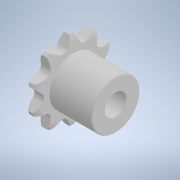
# Autodesk Inventor part: 25B10_()
Saved by Autodesk Inventor 2021 (Build 250183000, 183)
## iProperties
Created: 2025-03-15
Part Number: 25B10_()
Material: Generic
Catalog Web Link: www.cadenas.de
Description: K25B-Un-finished
Vendor: KANA
Document SubType Name: Modeling
Designer: psAdmin
Manufacturer: KANA
Mass: 2.29854 g
Surface Area: 15.9222 cm^2
Volume: 2.29854 cm^3
Density: 1 g/cm^3
Appearance: PSOLRGB-175-175-175
Category: PARTsolutions
Company: KANA
Title: K25B10
Author: Cadenas PARTsolutions
Comments: Un-finished
PSOL_IDENT_0: {$CADENAS_DATA/23d-libs/kana/sprockets/chain_no_25/un_finished_sprocket_steel/b_type/k25b.prj},157 {
PSOL_IDENT_1: VTYP=3D},{NB=25B10_()},{LINA=K25B10},{NN=K25B},{DATE=27.06.2023 01:46:12},{GEOMDATE=02.10.2020 05:05
PSOL_IDENT_2: :35},{VERSION=},{LINEID=10},{WBVAR=SURFT},{WBNUMERIC=}  {NB=25B10_()},{LINA=K25B10},{KT=DUMMY},{ORDE
PSOL_IDENT_3: RNO=K25B10},{TYPE=K25B},{NOT=10},{NOTX=10.000},{DP=20.55},{DO=23},{DC=17.25},{DC2=17.25},{T=2.8},{DR=
PSOL_IDENT_4: 3.3},{MAT=None},{MATC=},{SHAPE=C : Cutting type},{SHAPENB=C},{SD=6},{SURFT=},{SURFTNB=},{BD=14},{BL=
PSOL_IDENT_5: 15},{GD=0},{GDX=0},{S=0},{X=0},{VS=0},{SVDEL1=12},{SVDEL4=4},{SVDEL5=52},{DCX2=0},{CAUTION=The tooth
PSOL_IDENT_6: profile in the CAD models differ from the actual shape.}
NB: 25B10_()
NN: K25B
NT: Un-finished
NBSYN: 25B$NOT._($SURFT.)
LINA: K25B10
CATALOG: KANA
TYPE: K25B
NOT: 10
DP: 20.55
DO: 23
DC: 17.25
DC2: 17.25
T: 2.8
SHAPE: C : Cutting type
SD: 6
SURFT: No symbol : No
CAUTION: The tooth profile in the CAD models differ from the actual shape.
SUPPLIER: KANA
ARTICLENO: 25B10_()
BOMINFO: K25B10
CREATOR: CADENAS GmbH
Autodesk Inventor part; units mm, degrees
sketch "Sketch_4" plane through (0, 0, 0) normal (0, 0, 1) x (1, 0, 0)
  line L0 (15, 0) -> (0, 0)
  line L1 (0, 3.198) -> (0.198, 3)
  line L2 (0.198, 3) -> (14.802, 3)
  line L3 (14.802, 3) -> (15, 3.198)
  line L4 (15, 3.198) -> (15, 6.802)
  line L5 (15, 6.802) -> (14.802, 7)
  line L6 (14.802, 7) -> (2.8, 7)
  line L7 (2.8, 7) -> (2.8, 9.8274)
  arc A0 (2.8, 9.8274) -> (2.1, 11.5) centre (-0.477, 9.4387) ccw
  line L8 (2.1, 11.5) -> (0.7, 11.5)
  arc A1 (0.7, 11.5) -> (0, 9.8274) centre (3.277, 9.4387) ccw
  line L9 (0, 9.8274) -> (0, 3.198)
  constraints: 20 end point, 4 point on circle, 2 centre point
revolve "Revolution1" add sketch "Sketch_4" angle 360 about axis through (15, 0, 0) along (1, 0, 0)
sketch "Sketch_7" plane through (1.4, 0, 0) normal (1, 0, 0) x (0, 0, -1)
  circle A0 centre (0, 0) radius 15.3333
  line L0 (-11.0813, 3.0748) -> (-9.1281, 1.1862)
  arc A1 (-9.1281, -1.1862) -> (-9.1281, 1.1862) centre (-10.275, 0) ccw
  line L1 (-9.1281, -1.1862) -> (-11.0813, -3.0748)
  arc A2 (-11.0813, -3.0748) -> (-10.7723, -4.0259) centre (0, 0) ccw
  line L2 (-10.7723, -4.0259) -> (-8.082, -4.4057)
  arc A3 (-6.6875, -6.325) -> (-8.082, -4.4057) centre (-8.3126, -6.0395) ccw
  line L3 (-6.6875, -6.325) -> (-7.1576, -9.001)
  arc A4 (-7.1576, -9.001) -> (-6.3486, -9.5888) centre (0, 0) ccw
  line L4 (-6.3486, -9.5888) -> (-3.9489, -8.3148)
  arc A5 (-1.6926, -9.0479) -> (-3.9489, -8.3148) centre (-3.1751, -9.7721) ccw
  line L5 (-1.6926, -9.0479) -> (-0.5, -11.4891)
  arc A6 (-0.5, -11.4891) -> (0.5, -11.4891) centre (0, 0) ccw
  line L6 (0.5, -11.4891) -> (1.6926, -9.0479)
  arc A7 (3.9489, -8.3148) -> (1.6926, -9.0479) centre (3.1751, -9.7721) ccw
  line L7 (3.9489, -8.3148) -> (6.3486, -9.5888)
  arc A8 (6.3486, -9.5888) -> (7.1576, -9.001) centre (0, 0) ccw
  line L8 (7.1576, -9.001) -> (6.6875, -6.325)
  arc A9 (8.082, -4.4057) -> (6.6875, -6.325) centre (8.3126, -6.0395) ccw
  line L9 (8.082, -4.4057) -> (10.7723, -4.0259)
  arc A10 (10.7723, -4.0259) -> (11.0813, -3.0748) centre (0, 0) ccw
  line L10 (11.0813, -3.0748) -> (9.1281, -1.1862)
  arc A11 (9.1281, 1.1862) -> (9.1281, -1.1862) centre (10.275, 0) ccw
  line L11 (9.1281, 1.1862) -> (11.0813, 3.0748)
  arc A12 (11.0813, 3.0748) -> (10.7723, 4.0259) centre (0, 0) ccw
  line L12 (10.7723, 4.0259) -> (8.082, 4.4057)
  arc A13 (6.6875, 6.325) -> (8.082, 4.4057) centre (8.3126, 6.0395) ccw
  line L13 (6.6875, 6.325) -> (7.1576, 9.001)
  arc A14 (7.1576, 9.001) -> (6.3486, 9.5888) centre (0, 0) ccw
  line L14 (6.3486, 9.5888) -> (3.9489, 8.3148)
  arc A15 (1.6926, 9.0479) -> (3.9489, 8.3148) centre (3.1751, 9.7721) ccw
  line L15 (1.6926, 9.0479) -> (0.5, 11.4891)
  arc A16 (0.5, 11.4891) -> (-0.5, 11.4891) centre (0, 0) ccw
  line L16 (-0.5, 11.4891) -> (-1.6926, 9.0479)
  arc A17 (-3.9489, 8.3148) -> (-1.6926, 9.0479) centre (-3.1751, 9.7721) ccw
  line L17 (-3.9489, 8.3148) -> (-6.3486, 9.5888)
  arc A18 (-6.3486, 9.5888) -> (-7.1576, 9.001) centre (0, 0) ccw
  line L18 (-7.1576, 9.001) -> (-6.6875, 6.325)
  arc A19 (-8.082, 4.4057) -> (-6.6875, 6.325) centre (-8.3126, 6.0395) ccw
  line L19 (-8.082, 4.4057) -> (-10.7723, 4.0259)
  arc A20 (-10.7723, 4.0259) -> (-11.0813, 3.0748) centre (0, 0) ccw
  constraints: 40 end point, 40 point on circle, 21 centre point
extrude "Extrusion1" cut sketch "Sketch_7" along normal mid plane 3.2
ref_plane "body_XY" through (0, 0, 0) normal (1, 0, 0) x (0, 0, -1)
ref_plane "body_YZ" through (0, 0, 0) normal (0, 0, -1) x (0, 1, 0)
ref_plane "body_ZX" through (0, 0, 0) normal (0, 1, 0) x (1, 0, 0)
body "Solid1"
